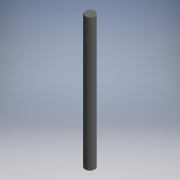
# Autodesk Inventor part: 2608532 EAGF-100-100-KF---(FST)
Saved by Autodesk Inventor 2017.3 (Build 213256000, 256)
## iProperties
Part Number: 2608532 EAGF-100-100-KF---(FST)
Material: Generic
Catalog Web Link: www.cadenas.de
Description: FENG-(FST)-Fuehrungsstange
Vendor: FESTO
Document SubType Name: Modeling
Designer: partserver
Manufacturer: FESTO
Mass: 166.478 g
Surface Area: 285.693 cm^2
Volume: 166.478 cm^3
Density: 1 g/cm^3
Appearance: PSOLRGB-128-128-128
Category: PARTsolutions
Company: FESTO
Title: 2608532 EAGF-100-100-KF---(FST)
Author: Cadenas PARTsolutions
Comments: Fuehrungsstange
PSOL_IDENT_0: {$CADENAS_DATA\23d-libs\festo\parts\e\eagf\parts\eagf_stange.prj},212 {VTYP=3D},{NB=2608532 EAGF-100
PSOL_IDENT_1: -100-KF---(FST)},{LINA=2608532 EAGF-100-100-KF---(FST)},{NN=FENG-(FST)},{DATE=20.07.2020 13:53:58},{
PSOL_IDENT_2: GEOMDATE=17.05.2016 07:24:00},{VERSION=},{LINEID=30},{WBVAR=HUB},{WBNUMERIC=HUB}  {NB=2608532 EAGF-1
PSOL_IDENT_3: 00-100-KF---(FST)},{LINA=2608532 EAGF-100-100-KF---(FST)},{KT=DUMMY},{TNR=2608532},{TYP=EAGF},{KDM=1
PSOL_IDENT_4: 00},{HUB=100},{D1=25.000},{D2=12.000},{T1=16.000},{T2=22.000},{L=243.000},{L1=343}
NB: 2608532 EAGF-100-100-KF---(FST)
NN: FENG-(FST)
NT: Fuehrungsstange
NBSYN: $TNR. $TYP.-$KDM.-$HUB.-KF---(FST)
LINA: 2608532 EAGF-100-100-KF---(FST)
CATALOG: Festo
TNR: 2608532
TYP: EAGF
KDM: 100
HUB: 100
D1: 25
D2: 12
T1: 16
T2: 22
L: 243
L1: 343
SUPPLIER: FESTO
ARTICLENO: 2608532 EAGF-100-100-KF---(FST)
BOMINFO: 2608532 EAGF-100-100-KF---(FST)
CREATOR: CADENAS GmbH
Autodesk Inventor part; units mm, degrees
sketch "Sketch_1" plane through (0, 0, 0) normal (1, 0, 0) x (0, 1, 0)
  line L0 (0, -343) -> (0, -24.9174)
  line L1 (0, -24.9174) -> (5.053, -22)
  line L2 (5.053, -22) -> (5.053, -0.947)
  line L3 (5.053, -0.947) -> (6, 0)
  line L4 (6, 0) -> (12.5, 0)
  line L5 (12.5, 0) -> (12.5, -341)
  line L6 (12.5, -341) -> (12.3399, -342.1392)
  arc A0 (11.3496, -343) -> (12.3399, -342.1392) centre (11.3496, -342) ccw
  line L7 (11.3496, -343) -> (0, -343)
  line L8 (0, -343) -> (0, -24.9174)
  constraints: 18 end point, 2 point on circle, 1 centre point
revolve "Revolution1" add sketch "Sketch_1" angle 360 about axis through (0, 0, -343) along (0, 0, -1)
thread "Thread1" size "M12x1.75" class "6H" standard "ISO Metric profile" length 15.053
ref_plane "ANBAU_XY" through (0, 0, 0) normal (0, 0, -1) x (1, 0, 0)
ref_plane "ANBAU_YZ" through (0, 0, 0) normal (1, 0, 0) x (0, -1, 0)
ref_plane "ANBAU_ZX" through (0, 0, 0) normal (0, -1, 0) x (0, 0, -1)
body "Solid1"
